Autodesk Fusion 360 part; units mm, degrees
(part 2 of 2)
sketch "Sketch4 (3)" plane through (0, -4, 0) normal (0, 1, 0) x (-1, 0, 0) in component "BottomLid"
  line L0 (-58.1, 88) -> (-58.1, 90)
  line L1 (-58.1, 90) -> (-69, 90)
  line L2 (-69, 90) -> (-69, 22.5)
  line L3 (-69, 22.5) -> (0, 22.5)
  line L4 (0, 22.5) -> (0, 90)
  line L5 (0, 90) -> (-28, 90)
  line L6 (-28, 90) -> (-28, 80)
  line L7 (-28, 80) -> (-30.5, 80)
  line L8 (-30.5, 80) -> (-30.5, 70)
  line L9 (-30.5, 70) -> (-38.5, 70)
  line L10 (-38.5, 70) -> (-38.5, 80)
  line L11 (-38.5, 80) -> (-41, 80)
  line L12 (-41, 80) -> (-41, 90)
  line L13 (-41, 90) -> (-48.9, 90)
  line L14 (-48.9, 90) -> (-48.9, 88)
  line L15 (-48.9, 88) -> (-43, 88)
  line L16 (-43, 88) -> (-43, 65)
  line L17 (-43, 65) -> (-20, 65)
  line L18 (-20, 65) -> (-20, 61)
  line L19 (-20, 61) -> (-64, 61)
  line L20 (-64, 61) -> (-64, 60)
  line L21 (-64, 60) -> (-52, 60)
  line L22 (-52, 60) -> (-52, 55)
  line L23 (-52, 55) -> (-67, 55)
  line L24 (-67, 55) -> (-67, 65)
  line L25 (-67, 65) -> (-64, 65)
  line L26 (-64, 65) -> (-64, 88)
  line L27 (-64, 88) -> (-58.1, 88)
  circle A0 centre (-66.75, 30) radius 0.95
  circle A1 centre (-66, 82) radius 0.95
  circle A2 centre (-2.25, 30) radius 0.95
  circle A3 centre (-3, 82) radius 0.95
  circle A4 centre (-41, 75) radius 0.95
  line L28 (-20, 65) -> (-30.5, 65)
  line L29 (-30.5, 65) -> (-30.5, 77)
  line L30 (-30.5, 77) -> (-20, 77)
  line L31 (-20, 77) -> (-20, 65)
  line L32 (-38.5, 70) -> (-38.5, 65)
  dimension "d287" = 12
  constraint horizontal L28
  constraint vertical L29
  constraint horizontal L30
  constraint vertical L31
  constraint coincident L17.end L18.start
  constraint coincident L9.end L10.start
  constraint coincident L17 L32.end
  constraint perpendicular L17 L32
  measures "d287" distance of L17.end L30.end
extrude "Extrude4'" cut sketch "Sketch4 (3)" against normal blind 1 contours L8 L17 L28 L29 L30 L31 | L9 L17 L29 L32 bodies 3 in component "BottomLid"
extrude "Extrude25" add 3 faces at (2, -2.6667, 2) (2, -2.6667, 18) (2, -2.6667, 42.6667) along direction (1, 0, 0) blind 2.5 on bodies 1 bodies 1 in component "BottomPart"
extrude "Extrude26" add 2 faces at (67, -2.6667, 22) (67, -2.6667, 4) along direction (-1, 0, 0) blind 2.5 on bodies 1 bodies 1 in component "BottomPart"
extrude "Extrude15'" add 2 faces at (67, -2.6667, -3.6667) (67, -1.3333, -23.1667) along direction (-1, 0, 0) blind 2.5 on bodies 2 bodies 2 in component "TopPart"
extrude "Extrude16" add 2 faces at (2, -2.6667, -3.6667) (2, -2.6667, -27.3333) along direction (1, 0, 0) blind 2.5 on bodies 2 bodies 2 in component "TopPart"
fillet "Fillet5" radius 2 5 edges at (20, -2, 61) (20, -2, 78) (39, -2, 78) (43, -2, 65) (39, -2, 65) on bodies 1 in component "BottomPart"
fillet "Fillet2" radius 8 2 edges at (69, 3.5, 90) (0, 3.5, 90) on bodies 1 in component "BottomPart"
fillet "Fillet1''" radius 8 2 edges at (69, -5, 90) (0, -5, 90) on bodies 3 in component "BottomLid"
fillet "Fillet3" radius 3 2 edges at (28, 3.5, 90) (41, 3.5, 90) on bodies 1 in component "BottomPart"
fillet "Fillet4" radius 2 2 edges at (41, -1.75, 80) (28, -1.75, 80) on bodies 1 in component "BottomPart"
fillet "Fillet2'" radius 3 2 edges at (28, -5, 90) (41, -5, 90) on bodies 3 in component "BottomLid"
fillet "Fillet3'" radius 2 2 edges at (28, -5, 80) (41, -5, 80) on bodies 3 in component "BottomLid"
fillet "Fillet4'" radius 2 14 edges at (38.75, -6, 80) (40.4142, -6, 80.5858) (41, -6, 84.5) (41.8787, -6, 89.1213) (52.5, -6, 90) (66.6569, -6, 87.6569) (69, -6, 52.25) (30.25, -6, 80) (28.5858, -6, 80.5858) (28, -6, 84.5) (27.1213, -6, 89.1213) (16.5, -6, 90) (2.3431, -6, 87.6569) (0, -6, 52.25) on bodies 3 in component "BottomLid"
fillet "Fillet6" radius 2 2 edges at (54, -2, 61) (62, -2, 61) on bodies 1 in component "BottomPart"
fillet "Fillet7" radius 1 5 edges at (34.25, 0, 60) (4.5, 0, 30) (67, 0, 49.5) (64.5, 0, 17) (65.75, 0, 34) on bodies 1 in component "BottomPart"
fillet "Fillet2''" radius 1 3 edges at (4.5, 0, -15.75) (34.5, 0, -31.5) (64.5, 0, -15.75) on bodies 2 in component "TopPart"
fillet "Fillet3''" radius 3 2 edges at (69, 3.5, -51.75) (0, 3.5, -51.75) on bodies 2 in component "TopPart"
fillet "Fillet4''" radius 2 5 edges at (69, 11, -35.375) (68.1213, 11, -50.8713) (34.5, 11, -51.75) (0.8787, 11, -50.8713) (0, 11, -24.375) on bodies 2 in component "TopPart"
fillet "Fillet8" radius 2 10 edges at (41, 11, 83.5) (41.8787, 11, 89.1213) (52.5, 11, 90) (66.6569, 11, 87.6569) (69, 11, 52.75) (28, 11, 83.5) (27.1213, 11, 89.1213) (16.5, 11, 90) (2.3431, 11, 87.6569) (0, 11, 41) on bodies 1 in component "BottomPart"
fillet "Fillet9" radius 3 4 edges at (68, 2.25, 59) (68, 2.25, 45) (68, 8.25, 45) (68, 8.25, 59) on bodies 1 in component "BottomPart"
fillet "Fillet10" radius 1 4 edges at (67, 0.5, 40) (54, 0.5, 80) (2, 0.5, 40) (15, 0.5, 80) on bodies 1 in component "BottomPart"
fillet "Fillet11" radius 5 1 edges at (68, 2.25, 23.5) on bodies 1 in component "BottomPart"
fillet "Fillet5'" radius 5 1 edges at (68, 2.25, -22) on bodies 2 in component "TopPart"
fillet "Fillet6'" radius 2 5 edges at (66.25, 11, -22) (68.4142, 10.4142, -22) (69, 8.125, -22) (69, 3.7145, -20.5355) (69, 2.25, -8.5) on bodies 2 in component "TopPart"
fillet "Fillet12" radius 2 5 edges at (66.25, 11, 23.5) (68.4142, 10.4142, 23.5) (69, 8.125, 23.5) (69, 3.7145, 22.0355) (69, 2.25, 9.25) on bodies 1 in component "BottomPart"
fillet "Fillet7'" radius 1 2 edges at (6.7369, 3.9843, -51.75) (6.7369, 6.5157, -49.75) on bodies 2 in component "TopPart"
fillet "Fillet1'''" radius 3 2 edges at (0, -5, -51.75) (69, -5, -51.75) on bodies 4 in component "TopLid"
fillet "Fillet2'''" radius 2 9 edges at (43, -6, -48.3481) (19.9019, -6, -40.25) (43, -6, -32.1519) (66.0981, -6, -40.25) (0, -6, -13.125) (0.8787, -6, -50.8713) (34.5, -6, -51.75) (68.1213, -6, -50.8713) (69, -6, -13.125) on bodies 4 in component "TopLid"
hole "Hole1" at (66.75, -6, 30) direction (0, 1, 0) diameter 4 depth 0.5 tip angle 118 bodies 3 in component "BottomLid"
hole "Hole2" at (66, -6, 82) direction (0, 1, 0) diameter 4 depth 0.5 tip angle 118 bodies 3 in component "BottomLid"
hole "Hole3" at (41, -6, 75) direction (0, 1, 0) diameter 4 depth 0.5 tip angle 118 bodies 3 in component "BottomLid"
hole "Hole4" at (3, -6, 82) direction (0, 1, 0) diameter 4 depth 0.5 tip angle 118 bodies 3 in component "BottomLid"
hole "Hole5" at (2.25, -6, 30) direction (0, 1, 0) diameter 4 depth 0.5 tip angle 118 bodies 3 in component "BottomLid"
hole "Hole1'" at (2.25, -6, 10) direction (0, 1, 0) diameter 4 depth 0.5 tip angle 118 bodies 4 in component "TopLid"
hole "Hole2'" at (2.25, -6, -15) direction (0, 1, 0) diameter 4 depth 0.5 tip angle 118 bodies 4 in component "TopLid"
hole "Hole3'" at (12, -6, -41.75) direction (0, 1, 0) diameter 4 depth 0.5 tip angle 118 bodies 4 in component "TopLid"
hole "Hole4'" at (66.75, -6, -15) direction (0, 1, 0) diameter 4 depth 0.5 tip angle 118 bodies 4 in component "TopLid"
hole "Hole5'" at (66.75, -6, 10) direction (0, 1, 0) diameter 4 depth 0.5 tip angle 118 bodies 4 in component "TopLid"
fillet "Fillet13" radius 1 8 edges at (69, 8.25, 52) (69, 5.25, 59) (69, 2.25, 52) (69, 5.25, 45) (67, 2.25, 52) (67, 5.25, 59) (67, 8.25, 52) (67, 5.25, 45) on bodies 1 in component "BottomPart"
fillet "Fillet14" radius 1 2 edges at (48.9, -1.5, 89) (58.1, -1.5, 89) on bodies 1 in component "BottomPart"
fillet "Fillet5''" radius 1 2 edges at (48.9, -5.5, 88.6614) (58.1, -5.5, 88.6614) on bodies 3 in component "BottomLid"
fillet "Fillet8'" radius 1 3 edges at (2, 0.5, -24.875) (34.5, 0.5, -49.75) (67, 0.5, -24.875) on bodies 2 in component "TopPart"
chamfer "Chamfer1" distance 0.95 angle 45 7 edges at (65.8643, 0, 29.6565) (65.8643, 0, 9.6565) (1.3643, 0, 9.6565) (1.3643, 0, 29.6565) (2.1143, -1.5, 82.3435) (40.1143, 0, 74.6565) (65.1143, 0, 81.6565) on bodies 1 in component "BottomPart"
chamfer "Chamfer1'" distance 0.95 angle 45 3 edges at (1.3643, 0, -15.3435) (11.1143, -1.5, -41.4065) (65.8643, 0, -15.3435) on bodies 2 in component "TopPart"
component "BottomPart" placed x (1, 0, 0) y (0, 1, 0) z (0, 0, 1) at (0, 0, 0)
component "TopPart" placed x (1, 0, 0) y (0, 1, 0) z (0, 0, 1) at (0, 0, 0)
component "BottomLid" placed x (1, 0, 0) y (0, 1, 0) z (0, 0, 1) at (0, 0, 0) in component "BottomPart"
component "TopLid" placed x (1, 0, 0) y (0, 1, 0) z (0, 0, 1) at (0, 0, 0) in component "TopPart"
equation "d219 = ( 9.2 / 2 ) * 1 mm"
equation "d248 = 1.25 mm + ( 7 / 2 ) * 1 mm"
